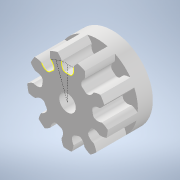
# Autodesk Inventor part: SmallGear9T
Saved by Autodesk Inventor 2022 (Build 260153070, 153G)
## iProperties
Created: 2021-11-03
Part Number: SmallGear9T
Material: Generic
Document SubType Name: Modeling
Designer: a laptop
Density: 1 g/cm^3
Appearance: Default
Author: a laptop
Autodesk Inventor part; units mm, degrees
ref_plane "YZ Plane" through (0, 0, 0) normal (1, 0, 0) x (0, 1, 0)
ref_plane "XZ Plane" through (0, 0, 0) normal (0, 1, 0) x (-1, 0, 0)
ref_plane "XY Plane" through (0, 0, 0) normal (0, 0, 1) x (1, 0, 0)
sketch "Sketch1" plane through (0, 0, 0) normal (0, 0, 1) x (1, 0, 0)
  spline S0 degree 3 poles (-1.3464, 5.2146) (-1.2887, 5.1626) (-1.1733, 5.0587) (-1.0189, 4.8841) (-0.8785, 4.6973) (-0.8096, 4.558) (-0.7752, 4.4884) knots 0 0 0 0 0.250071 0.500149 0.750165 1 1 1 1
  spline S1 degree 3 poles (-0.7752, 4.4884) (-0.7857, 4.4211) (-0.8066, 4.2867) (-0.8068, 4.0817) (-0.7737, 3.8799) (-0.7064, 3.686) (-0.5864, 3.5181) (-0.4401, 3.4219) (-0.3061, 3.3934) (-0.1697, 3.3977) (0, 3.4077) (0.1697, 3.3977) (0.3061, 3.3934) (0.4401, 3.4219) (0.5864, 3.5181) (0.7064, 3.686) (0.7737, 3.8799) (0.8068, 4.0817) (0.8066, 4.2867) (0.7857, 4.4211) (0.7752, 4.4884) knots 0 0 0 0 0.062606 0.125231 0.187814 0.250234 0.312597 0.374754 0.406093 0.437398 0.5 0.562602 0.593907 0.625246 0.687403 0.749766 0.812186 0.874769 0.937394 1 1 1 1
  spline S2 degree 3 poles (0.7752, 4.4884) (0.8096, 4.558) (0.8785, 4.6973) (1.0189, 4.8841) (1.1733, 5.0587) (1.2887, 5.1626) (1.3464, 5.2146) knots 0 0 0 0 0.249835 0.499851 0.749929 1 1 1 1
  circle A0 centre (0, 0) radius 3.4037 construction
  circle A1 centre (0, 0) radius 4.4316 construction
  circle A2 centre (0, 0) radius 4.5 construction
  circle A3 centre (0, 0) radius 5.3856
  point P0 (-1.1764, 5.0556)
  point P1 (-1.0212, 4.882)
  point P2 (-0.8847, 4.6936)
  point P3 (-0.8014, 4.2861)
  point P4 (-0.8012, 4.0821)
  point P5 (-0.7679, 3.881)
  point P6 (-0.6976, 3.6902)
  point P7 (-0.577, 3.5267)
  point P8 (-0.4056, 3.4189)
  point P9 (-0.3058, 3.3975)
  point P10 (-0.2038, 3.3969)
  point P11 (0, 3.4037)
  point P12 (0.2038, 3.3969)
  point P13 (0.3058, 3.3975)
  point P14 (0.4056, 3.4189)
  point P15 (0.577, 3.5267)
  point P16 (0.6976, 3.6902)
  point P17 (0.7679, 3.881)
  point P18 (0.8012, 4.0821)
  point P19 (0.8014, 4.2861)
  point P20 (0.8847, 4.6936)
  point P21 (1.0212, 4.882)
  point P22 (1.1764, 5.0556)
  constraints: 4 centre point, 2 point on circle, 61 other
extrude "Extrusion1" add sketch "Sketch1" against normal blind 3
extrude "Extrusion2" cut sketch "Sketch1" against normal blind 10 contours A3 S2 S1 S0 picked at (0.151, 4.7811)
pattern_circular "Circular Pattern1" count 9 over 360 about axis through (0, 0, 0) along (0, 0, -1) of "Extrusion2"
sketch "Sketch2" plane through (0, 0, 0) normal (0, 0, 1) x (1, 0, 0)
  line L0 (-2.2912, 3.9366) -> (-0.7752, 4.4884) construction
  line L1 (0.7752, 4.4884) -> (-0.7752, 4.4884) construction
  line L2 (-1.5332, 4.2125) -> (0, 0) construction
  line L3 (0, 0) -> (0, 4.4884) construction
  constraints: 8 end point, 2 midpoint, 1 horizontal, 1 horizontal alignment, 1 other
sketch "Sketch3" plane through (0, 0, 0) normal (0, 0, 1) x (1, 0, 0)
  circle A0 centre (0, 0) radius 1.1
  dimension "d7" = 2.2
  constraints: 1 centre point, 1 coincident
  measures "d7" diameter of A0
extrude "Extrusion3" cut sketch "Sketch3" against normal blind 3
sketch "Sketch4" plane through (0, 0, -3) normal (0, 0, -1) x (-1, 0, 0)
  spline S0 degree 3 poles (4.3833, 3.1292) (4.2345, 3.124) (4.1103, 3.1196) (3.7176, 3.0447) (3.6285, 3.0057) (3.4789, 2.94) knots 0 0 0 0 0.483183 0.483183 1 1 1 1
  spline S1 degree 3 poles (3.4789, 2.94) (3.4071, 2.8211) (3.3199, 2.6768) (3.1107, 2.4977) (3.0126, 2.4192) (2.8175, 2.3439) (2.7412, 2.3282) (2.6114, 2.3305) (2.5511, 2.3393) (2.4341, 2.39) (2.3938, 2.4228) (2.3328, 2.477) (2.0303, 2.7209) (1.9226, 2.8253) (1.8877, 2.8686) (1.84, 2.9802) (1.8263, 3.0373) (1.8195, 3.1506) (1.8216, 3.2234) (1.878, 3.421) (1.9296, 3.5182) (2.0754, 3.748) (2.1906, 3.8487) (2.2912, 3.9366) knots 0 0 0 0 0.483096 0.483096 0.641744 0.641744 0.734426 0.734426 0.798163 0.798163 0.858409 0.858409 0.904001 0.904001 0.923629 0.923629 0.939466 0.939466 0.952503 0.952503 0.967089 0.967089 1 1 1 1
  spline S2 degree 3 poles (2.2912, 3.9366) (2.3299, 4.0953) (2.3529, 4.1898) (2.3585, 4.5896) (2.3412, 4.7126) (2.3205, 4.8601) knots 0 0 0 0 0.516817 0.516817 1 1 1 1
  arc A0 (2.3205, 4.8601) -> (1.3464, 5.2146) centre (0, 0) ccw
  spline S3 degree 3 poles (1.3464, 5.2146) (1.2357, 5.115) (1.1434, 5.0318) (0.8907, 4.722) (0.8476, 4.6349) (0.7752, 4.4884) knots 0 0 0 0 0.483183 0.483183 1 1 1 1
  spline S4 degree 3 poles (0.7752, 4.4884) (0.7966, 4.3511) (0.8226, 4.1845) (0.7775, 3.9129) (0.7527, 3.7897) (0.6517, 3.6065) (0.6033, 3.5456) (0.5024, 3.4638) (0.4506, 3.4319) (0.3283, 3.3955) (0.2764, 3.3946) (0.1949, 3.397) (-0.1936, 3.3893) (-0.3432, 3.4001) (-0.3979, 3.4108) (-0.5061, 3.4657) (-0.5533, 3.5007) (-0.6314, 3.5831) (-0.6766, 3.6401) (-0.7603, 3.8278) (-0.7833, 3.9354) (-0.8194, 4.2052) (-0.7958, 4.3564) (-0.7752, 4.4884) knots 0 0 0 0 0.483096 0.483096 0.641744 0.641744 0.734426 0.734426 0.798163 0.798163 0.858409 0.858409 0.904001 0.904001 0.923629 0.923629 0.939466 0.939466 0.952503 0.952503 0.967089 0.967089 1 1 1 1
  spline S5 degree 3 poles (-0.7752, 4.4884) (-0.8476, 4.6349) (-0.8907, 4.722) (-1.1434, 5.0318) (-1.2357, 5.115) (-1.3464, 5.2146) knots 0 0 0 0 0.516817 0.516817 1 1 1 1
  arc A1 (-1.3464, 5.2146) -> (-2.3205, 4.8601) centre (0, 0) ccw
  spline S6 degree 3 poles (-2.3205, 4.8601) (-2.3412, 4.7126) (-2.3585, 4.5896) (-2.3529, 4.1898) (-2.3299, 4.0953) (-2.2912, 3.9366) knots 0 0 0 0 0.483183 0.483183 1 1 1 1
  spline S7 degree 3 poles (-2.2912, 3.9366) (-2.1866, 3.8452) (-2.0596, 3.7342) (-1.9195, 3.4972) (-1.8594, 3.3869) (-1.819, 3.1817) (-1.8169, 3.1039) (-1.8416, 2.9764) (-1.8608, 2.9186) (-1.931, 2.8121) (-1.9703, 2.7781) (-2.0343, 2.7275) (-2.327, 2.4719) (-2.4485, 2.384) (-2.4972, 2.3571) (-2.6155, 2.3296) (-2.6741, 2.326) (-2.7868, 2.339) (-2.8581, 2.3536) (-3.0429, 2.4435) (-3.1297, 2.5112) (-3.3307, 2.6947) (-3.4098, 2.8257) (-3.4789, 2.94) knots 0 0 0 0 0.483096 0.483096 0.641744 0.641744 0.734426 0.734426 0.798163 0.798163 0.858409 0.858409 0.904001 0.904001 0.923629 0.923629 0.939466 0.939466 0.952503 0.952503 0.967089 0.967089 1 1 1 1
  spline S8 degree 3 poles (-3.4789, 2.94) (-3.6285, 3.0057) (-3.7176, 3.0447) (-4.1103, 3.1196) (-4.2345, 3.124) (-4.3833, 3.1292) knots 0 0 0 0 0.516817 0.516817 1 1 1 1
  arc A2 (-4.3833, 3.1292) -> (-4.9016, 2.2314) centre (0, 0) ccw
  spline S9 degree 3 poles (-4.9016, 2.2314) (-4.8227, 2.1052) (-4.7568, 1.9998) (-4.4956, 1.6972) (-4.4172, 1.6396) (-4.2856, 1.5428) knots 0 0 0 0 0.483183 0.483183 1 1 1 1
  spline S10 degree 3 poles (-4.2856, 1.5428) (-4.1467, 1.5401) (-3.9781, 1.5367) (-3.7184, 1.4452) (-3.6014, 1.3993) (-3.4386, 1.2681) (-3.3869, 1.2099) (-3.324, 1.0963) (-3.3015, 1.0397) (-3.2869, 0.913) (-3.2951, 0.8617) (-3.3115, 0.7818) (-3.3715, 0.3979) (-3.4081, 0.2524) (-3.4281, 0.2005) (-3.501, 0.1034) (-3.5436, 0.063) (-3.6383, 0.0004) (-3.7023, -0.0342) (-3.9017, -0.0841) (-4.0116, -0.088) (-4.2836, -0.0767) (-4.4284, -0.0272) (-4.5548, 0.016) knots 0 0 0 0 0.483096 0.483096 0.641744 0.641744 0.734426 0.734426 0.798163 0.798163 0.858409 0.858409 0.904001 0.904001 0.923629 0.923629 0.939466 0.939466 0.952503 0.952503 0.967089 0.967089 1 1 1 1
  spline S11 degree 3 poles (-4.5548, 0.016) (-4.7116, -0.0299) (-4.805, -0.0572) (-5.1539, -0.2523) (-5.2518, -0.3288) (-5.3692, -0.4204) knots 0 0 0 0 0.516817 0.516817 1 1 1 1
  arc A3 (-5.3692, -0.4204) -> (-5.1892, -1.4413) centre (0, 0) ccw
  spline S12 degree 3 poles (-5.1892, -1.4413) (-5.0476, -1.4873) (-4.9294, -1.5257) (-4.5348, -1.5896) (-4.4377, -1.5834) (-4.2746, -1.5729) knots 0 0 0 0 0.483183 0.483183 1 1 1 1
  spline S13 degree 3 poles (-4.2746, -1.5729) (-4.1665, -1.4857) (-4.0352, -1.3799) (-3.7774, -1.2831) (-3.6583, -1.243) (-3.4492, -1.2389) (-3.3722, -1.2503) (-3.251, -1.2968) (-3.1974, -1.3257) (-3.1047, -1.4134) (-3.0781, -1.4579) (-3.0393, -1.5297) (-2.8384, -1.8624) (-2.773, -1.9973) (-2.7549, -2.05) (-2.7483, -2.1712) (-2.755, -2.2295) (-2.7874, -2.3383) (-2.8142, -2.406) (-2.9348, -2.5724) (-3.0165, -2.6461) (-3.2321, -2.8122) (-3.3749, -2.8674) (-3.4994, -2.9155) knots 0 0 0 0 0.483096 0.483096 0.641744 0.641744 0.734426 0.734426 0.798163 0.798163 0.858409 0.858409 0.904001 0.904001 0.923629 0.923629 0.939466 0.939466 0.952503 0.952503 0.967089 0.967089 1 1 1 1
  spline S14 degree 3 poles (-3.4994, -2.9155) (-3.5901, -3.0515) (-3.644, -3.1324) (-3.786, -3.5061) (-3.8118, -3.6277) (-3.8428, -3.7733) knots 0 0 0 0 0.516817 0.516817 1 1 1 1
  arc A4 (-3.8428, -3.7733) -> (-3.0487, -4.4397) centre (0, 0) ccw
  spline S15 degree 3 poles (-3.0487, -4.4397) (-2.9106, -4.3838) (-2.7955, -4.3373) (-2.452, -4.1326) (-2.3817, -4.0654) (-2.2636, -3.9526) knots 0 0 0 0 0.483183 0.483183 1 1 1 1
  spline S16 degree 3 poles (-2.2636, -3.9526) (-2.2367, -3.8163) (-2.2041, -3.6508) (-2.0689, -3.411) (-2.0035, -3.3037) (-1.8459, -3.1661) (-1.7796, -3.1254) (-1.6568, -3.0831) (-1.5972, -3.0708) (-1.4699, -3.0784) (-1.4208, -3.0954) (-1.345, -3.1255) (-0.9773, -3.2512) (-0.8404, -3.3125) (-0.7927, -3.3412) (-0.7097, -3.4298) (-0.6774, -3.4788) (-0.6322, -3.583) (-0.6092, -3.652) (-0.5947, -3.857) (-0.6099, -3.966) (-0.6683, -4.2318) (-0.7422, -4.3658) (-0.8067, -4.4828) knots 0 0 0 0 0.483096 0.483096 0.641744 0.641744 0.734426 0.734426 0.798163 0.798163 0.858409 0.858409 0.904001 0.904001 0.923629 0.923629 0.939466 0.939466 0.952503 0.952503 0.967089 0.967089 1 1 1 1
  spline S17 degree 3 poles (-0.8067, -4.4828) (-0.7887, -4.6452) (-0.778, -4.7419) (-0.6465, -5.1194) (-0.5882, -5.2291) (-0.5183, -5.3606) knots 0 0 0 0 0.516817 0.516817 1 1 1 1
  arc A5 (-0.5183, -5.3606) -> (0.5183, -5.3606) centre (0, 0) ccw
  spline S18 degree 3 poles (0.5183, -5.3606) (0.5882, -5.2291) (0.6465, -5.1194) (0.778, -4.7419) (0.7887, -4.6452) (0.8067, -4.4828) knots 0 0 0 0 0.483183 0.483183 1 1 1 1
  spline S19 degree 3 poles (0.8067, -4.4828) (0.7396, -4.3612) (0.6582, -4.2135) (0.6077, -3.9428) (0.5888, -3.8186) (0.6211, -3.6119) (0.6457, -3.5381) (0.7126, -3.4268) (0.7504, -3.379) (0.8528, -3.303) (0.9013, -3.2845) (0.9787, -3.2588) (1.3412, -3.1187) (1.4854, -3.0777) (1.5405, -3.0691) (1.661, -3.0836) (1.7173, -3.1003) (1.8188, -3.1511) (1.8807, -3.1892) (2.0237, -3.3369) (2.0821, -3.4302) (2.2082, -3.6713) (2.2378, -3.8215) (2.2636, -3.9526) knots 0 0 0 0 0.483096 0.483096 0.641744 0.641744 0.734426 0.734426 0.798163 0.798163 0.858409 0.858409 0.904001 0.904001 0.923629 0.923629 0.939466 0.939466 0.952503 0.952503 0.967089 0.967089 1 1 1 1
  spline S20 degree 3 poles (2.2636, -3.9526) (2.3817, -4.0654) (2.452, -4.1326) (2.7955, -4.3373) (2.9106, -4.3838) (3.0487, -4.4397) knots 0 0 0 0 0.516817 0.516817 1 1 1 1
  arc A6 (3.0487, -4.4397) -> (3.8428, -3.7733) centre (0, 0) ccw
  spline S21 degree 3 poles (3.8428, -3.7733) (3.8118, -3.6277) (3.786, -3.5061) (3.644, -3.1324) (3.5901, -3.0515) (3.4994, -2.9155) knots 0 0 0 0 0.483183 0.483183 1 1 1 1
  spline S22 degree 3 poles (3.4994, -2.9155) (3.3699, -2.8654) (3.2126, -2.8046) (2.9999, -2.6298) (2.9056, -2.5467) (2.7975, -2.3677) (2.7689, -2.2953) (2.7486, -2.167) (2.7468, -2.1062) (2.7764, -1.9821) (2.8016, -1.9367) (2.8444, -1.8673) (3.0321, -1.527) (3.1162, -1.4028) (3.1528, -1.3608) (3.2545, -1.2945) (3.3083, -1.2711) (3.4187, -1.2448) (3.4907, -1.2341) (3.6952, -1.2554) (3.7998, -1.2893) (4.0515, -1.393) (4.1706, -1.489) (4.2746, -1.5729) knots 0 0 0 0 0.483096 0.483096 0.641744 0.641744 0.734426 0.734426 0.798163 0.798163 0.858409 0.858409 0.904001 0.904001 0.923629 0.923629 0.939466 0.939466 0.952503 0.952503 0.967089 0.967089 1 1 1 1
  spline S23 degree 3 poles (4.2746, -1.5729) (4.4377, -1.5834) (4.5348, -1.5896) (4.9294, -1.5257) (5.0476, -1.4873) (5.1892, -1.4413) knots 0 0 0 0 0.516817 0.516817 1 1 1 1
  arc A7 (5.1892, -1.4413) -> (5.3692, -0.4204) centre (0, 0) ccw
  spline S24 degree 3 poles (5.3692, -0.4204) (5.2518, -0.3288) (5.1539, -0.2523) (4.805, -0.0572) (4.7116, -0.0299) (4.5548, 0.016) knots 0 0 0 0 0.483183 0.483183 1 1 1 1
  spline S25 degree 3 poles (4.5548, 0.016) (4.4233, -0.0289) (4.2637, -0.0835) (3.9884, -0.0862) (3.8628, -0.0832) (3.6649, -0.0155) (3.5965, 0.0215) (3.4984, 0.1067) (3.458, 0.1522) (3.4009, 0.2663) (3.3911, 0.3172) (3.3792, 0.398) (3.3042, 0.7793) (3.2889, 0.9284) (3.2899, 0.9841) (3.3252, 1.1003) (3.3514, 1.1528) (3.419, 1.244) (3.4673, 1.2984) (3.6376, 1.4135) (3.7396, 1.4548) (3.999, 1.5371) (4.152, 1.5402) (4.2856, 1.5428) knots 0 0 0 0 0.483096 0.483096 0.641744 0.641744 0.734426 0.734426 0.798163 0.798163 0.858409 0.858409 0.904001 0.904001 0.923629 0.923629 0.939466 0.939466 0.952503 0.952503 0.967089 0.967089 1 1 1 1
  spline S26 degree 3 poles (4.2856, 1.5428) (4.4172, 1.6396) (4.4956, 1.6972) (4.7568, 1.9998) (4.8227, 2.1052) (4.9016, 2.2314) knots 0 0 0 0 0.516817 0.516817 1 1 1 1
  arc A8 (4.9016, 2.2314) -> (4.3833, 3.1292) centre (0, 0) ccw
  constraints: 9 centre point, 72 other
extrude "Extrusion4" add sketch "Sketch4" along normal blind 1
sketch "Sketch5" plane through (0, 0, -4) normal (0, 0, -1) x (-1, 0, 0)
  circle A0 centre (0, 0) radius 3.05
  circle A1 centre (0, 0) radius 5.3856
  arc A2 (-0.5183, -5.3606) -> (0.5183, -5.3606) centre (0, 0) ccw projected
  dimension "d12" = 6.1
  constraints: 2 centre point, 2 concentric, 1 coincident
  measures "d12" diameter of A0
extrude "Extrusion5" add sketch "Sketch5" along normal blind 2
equation "\"d0\" = FaceWidth"
equation "\"Module\" = 1"
equation "\"PressureAngle\" = 10deg"
equation "\"UnitProfileClearance\" = 0.25"
equation "\"UnitRoundRadius\" = 0.3025"
equation "\"HeadDiameter\" = 10.77128"
equation "\"RootDiameter\" = 6.80735"
equation "\"BaseDiameter\" = 8.86327"
equation "\"PitchDiameter\" = 9"
equation "\"FaceWidth\" = 3"
equation "\"HelixAngle\" = 0"
equation "\"UnitCorrection\" = 0.153676"
equation "\"UnitAddendumModification\" = 0.268038"
equation "\"CircularPitch\" = 3.141593"
equation "\"UnitBacklashShift\" = 0"
equation "\"TotalToolShift\" = 0.15368"
equation "\"IsInternal\" = 0"
body "Solid1"
